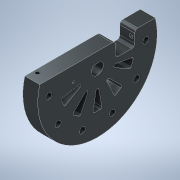
# Autodesk Inventor part: Capstondisc_v2
Saved by Autodesk Inventor 2022 (Build 260153000, 153)
## iProperties
Created: 2022-03-10
Part Number: Capstondisc_v2
Material: Generisch
Document SubType Name: Modeling
Designer: 123St
Density: 1 g/cm^3
Appearance: Eisen - Grau
SmallCapston_Thickness: 10,000 mm
CapstonV2_ShaftDia: 8,000 mm
Poligonprofil_Ausnehmung: 1,000 mm
Author: 123St
Autodesk Inventor part; units mm, degrees
ref_plane "YZ Plane" through (0, 0, 0) normal (1, 0, 0) x (0, 1, 0)
ref_plane "XZ Plane" through (0, 0, 0) normal (0, 1, 0) x (-1, 0, 0)
ref_plane "XY Plane" through (0, 0, 0) normal (0, 0, 1) x (1, 0, 0)
sketch "Skizze1" plane through (0, 0, 0) normal (1, 0, 0) x (0, 1, 0)
  arc A0 (10, 38.7298) -> (10, -38.7298) centre (0, 0) ccw
  line L0 (10, 38.7298) -> (10, -12)
  line L1 (10, -38.7298) -> (10, -25)
  line L2 (10, -12) -> (0, -12)
  line L3 (0, -12) -> (0, -25)
  line L4 (0, -25) -> (10, -25)
  circle A1 centre (0, 32.5) radius 2
  circle A2 centre (-19.103, 26.2931) radius 2
  circle A3 centre (-30.9093, 10.0431) radius 2
  circle A4 centre (-30.9093, -10.0431) radius 2
  circle A5 centre (-19.103, -26.2931) radius 2
  circle A6 centre (0, -32.5) radius 2
  circle A7 centre (0, 0) radius 1.25
  line L5 (-7, 0) -> (-24.8022, 3.139)
  line L6 (-24.8022, 3.139) -> (-24.8022, -3.139)
  line L7 (-24.8022, -3.139) -> (-7, 0)
  line L8 (-54.5, 0) -> (47, 0) construction
  line L9 (-18.5163, -16.7972) -> (-5.7341, -4.015)
  line L10 (-5.7341, -4.015) -> (-22.1172, -11.6546)
  line L11 (-22.1172, -11.6546) -> (-18.5163, -16.7972)
  line L12 (-5.5331, -24.38) -> (-2.3941, -6.5778)
  line L13 (-2.3941, -6.5778) -> (-11.4325, -22.2328)
  line L14 (-11.4325, -22.2328) -> (-5.5331, -24.38)
  line L15 (-18.5163, 16.7972) -> (-5.7341, 4.015)
  line L16 (-5.7341, 4.015) -> (-22.1172, 11.6546)
  line L17 (-22.1172, 11.6546) -> (-18.5163, 16.7972)
  line L18 (-5.5331, 24.38) -> (-2.3941, 6.5778)
  line L19 (-2.3941, 6.5778) -> (-11.4325, 22.2328)
  line L20 (-11.4325, 22.2328) -> (-5.5331, 24.38)
  circle A8 centre (0, 0) radius 25 construction
  circle A9 centre (0, 0) radius 32.5 construction
  point P0 (-24.8022, 0)
  dimension "d50" = 65
  dimension "d0" = 80
  dimension "d3" = 10
  dimension "d4" = 10
  dimension "d5" = 10
  dimension "d7" = 0
  dimension "d8" = 4
  dimension "d11" = 180
  dimension "d13" = 2.5
  dimension "d19" = 20
  dimension "d22" = 0
  dimension "d23" = 7
  dimension "d26" = 70
  dimension "d49" = 50
  dimension "d51" = 12
  constraints: 40 end point, 9 centre point, 6 symmetric about line, 4 coincident, 4 point on circle, 3 vertical, 2 perpendicular, 1 horizontal, 1 midpoint, 1 point on line, 1 vertical alignment, 26 other
  measures "d0" diameter of A0
  measures "d3" distance from line of point (0, 0) L0
  measures "d4" distance from line of point (0, 0) L1
  measures "d5" distance of L3.end L1.end
  measures "d7" horizontal distance of point (0, 0) A1.centre
  measures "d8" diameter of A1
  measures "d13" diameter of A7
  measures "d19" angle of L7 L5
  measures "d22" distance from line of L8 L5.start
  measures "d23" distance of point (0, 0) L5.start
  measures "d49" diameter of A8
  measures "d51" distance between parallel lines of L8 L2
extrude "Extrusion1" add sketch "Skizze1" along normal blind 10
fillet "Rundung1" radius 1 15 edges at (5, -5.5331, -24.38) (5, -11.4325, -22.2328) (5, -18.5163, -16.7972) (5, -22.1172, -11.6546) (5, -24.8022, -3.139) (5, -24.8022, 3.139) (5, -18.5163, 16.7972) (5, -22.1172, 11.6546) (5, -11.4325, 22.2328) (5, -5.5331, 24.38) (5, -2.3941, 6.5778) (5, -5.7341, 4.015) (5, -7, 0) (5, -5.7341, -4.015) (5, -2.3941, -6.5778)
fillet "Rundung2" radius 2 4 edges at (5, 10, -12) (5, 0, -12) (5, 0, -25) (5, 10, -25)
sketch "Skizze2" plane through (10, 0, 0) normal (1, 0, 0) x (0, 0, -1)
  circle A0 centre (-16, 0) radius 0.75
  point P0 (0, 0)
  dimension "d30" = 1.5
  dimension "d31" = 16
  constraints: 1 centre point
  measures "d30" diameter of A0
  measures "d31" distance of point (0, 0) A0.centre
extrude "Extrusion2" cut sketch "Skizze2" against normal blind 10
sketch "Skizze3" plane through (0, 2, -25) normal (0, 0, 1) x (1, 0, 0)
  circle A0 centre (7.5, 3) radius 1.25
  line L0 (10, 6) -> (10, 0) projected
  line L1 (0, 6) -> (10, 6) projected
  point P0 (0, -2)
  point P1 (10, 0.8802)
  dimension "d35" = 2.5
  dimension "d36" = 2.5
  dimension "d37" = 3
  constraints: 1 centre point
  measures "d35" diameter of A0
  measures "d36" distance from line of L0 A0.centre
  measures "d37" distance from line of L1 A0.centre
extrude "Extrusion3" cut sketch "Skizze3" against normal blind 12
sketch "Skizze4" plane through (0, 10, 38.7298) normal (0, 1, 0) x (1, 0, 0)
  circle A0 centre (2.5, 6) radius 1.25
  line L0 (0, 48.7298) -> (0, 0) projected
  line L1 (0, 0) -> (10, 0) projected
  point P0 (0, 38.7298)
  dimension "d40" = 2.5
  dimension "d41" = 2.5
  dimension "d42" = 6
  constraints: 1 centre point
  measures "d40" diameter of A0
  measures "d41" distance from line of L0 A0.centre
  measures "d42" distance from line of L1 A0.centre
extrude "Extrusion4" cut sketch "Skizze4" against normal blind 10
sketch "Skizze5" plane through (10, 0, 0) normal (1, 0, 0) x (0, 0, -1)
  circle A0 centre (0, 0) radius 1.25 projected
  arc A1 (2.6458, -3) -> (-2.6458, -3) centre (0, 0) ccw
  line L0 (-2.6458, -3) -> (2.6458, -3)
  circle A2 centre (0, 0) radius 4
  line L1 (-2.6458, 3) -> (2.6458, 3)
  line L2 (0, 0) -> (0, 3) construction
  point P0 (-2.6458, -3)
  dimension "CapstonV2_ShaftDia" = 8
  dimension "Poligonprofil_Ausnehmung" = 1
  dimension "d52" = 1
  constraints: 6 end point, 5 point on circle, 2 centre point, 2 coincident, 2 horizontal, 1 midpoint
  measures "CapstonV2_ShaftDia" diameter of A1
  measures "Poligonprofil_Ausnehmung" distance edge to line of A1 L0
  measures "d52" distance edge to line of A1 L1
extrude "Extrusion5" cut sketch "Skizze5" against normal blind 10 contours L0 A1 L1 | A2 L0
equation "\"d50\" = 0.5 * d0 + 0.5 * d49"
